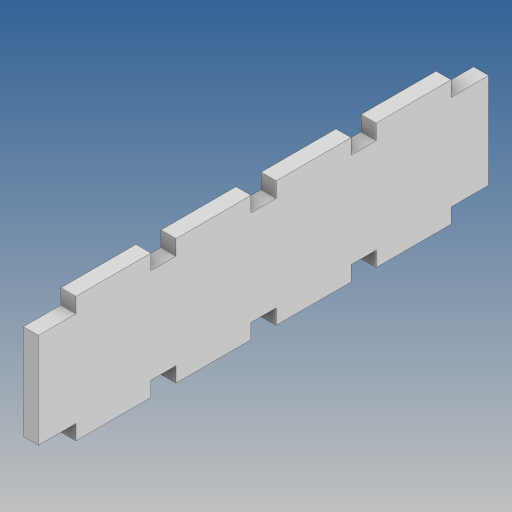
# Autodesk Inventor part: Pieza9
Saved by Autodesk Inventor 2024 (Build 280153000, 153)
## iProperties
Created: 2024-05-31
Part Number: Pieza9
Material: Genérico
Document SubType Name: Modeling
Designer: Pablo
Density: 1 g/cm^3
Appearance: Valor por defecto
Author: Pablo
Autodesk Inventor part; units mm, degrees
ref_plane "YZ Plane" through (0, 0, 0) normal (1, 0, 0) x (0, 1, 0)
ref_plane "XZ Plane" through (0, 0, 0) normal (0, 1, 0) x (-1, 0, 0)
ref_plane "XY Plane" through (0, 0, 0) normal (0, 0, 1) x (1, 0, 0)
sketch "Boceto1" plane through (0, 0, 0) normal (1, 0, 0) x (0, 1, 0)
  line L0 (0, 0) -> (19, 0)
  line L1 (19, 0) -> (19, -90)
  line L2 (19, -90) -> (0, -90)
  line L3 (0, -90) -> (0, 0)
  line L4 (19, -7.5) -> (22, -7.5)
  line L5 (22, -7.5) -> (22, -22.5)
  line L6 (22, -22.5) -> (19, -22.5)
  line L7 (19, -22.5) -> (19, -7.5)
  line L8 (19, -27.5) -> (22, -27.5)
  line L9 (22, -27.5) -> (22, -42.5)
  line L10 (22, -42.5) -> (19, -42.5)
  line L11 (19, -42.5) -> (19, -27.5)
  line L12 (19, -47.5) -> (22, -47.5)
  line L13 (22, -47.5) -> (22, -62.5)
  line L14 (22, -62.5) -> (19, -62.5)
  line L15 (19, -62.5) -> (19, -47.5)
  line L16 (19, -67.5) -> (22, -67.5)
  line L17 (22, -67.5) -> (22, -82.5)
  line L18 (22, -82.5) -> (19, -82.5)
  line L19 (19, -82.5) -> (19, -67.5)
  line L20 (9.5, 0) -> (9.5, -90) construction
  line L21 (0, -7.5) -> (-3, -7.5)
  line L22 (-3, -7.5) -> (-3, -22.5)
  line L23 (-3, -22.5) -> (0, -22.5)
  line L24 (0, -22.5) -> (0, -7.5)
  line L25 (0, -27.5) -> (-3, -27.5)
  line L26 (-3, -27.5) -> (-3, -42.5)
  line L27 (-3, -42.5) -> (0, -42.5)
  line L28 (0, -42.5) -> (0, -27.5)
  line L29 (0, -47.5) -> (-3, -47.5)
  line L30 (-3, -47.5) -> (-3, -62.5)
  line L31 (-3, -62.5) -> (0, -62.5)
  line L32 (0, -62.5) -> (0, -47.5)
  line L33 (0, -67.5) -> (-3, -67.5)
  line L34 (-3, -67.5) -> (-3, -82.5)
  line L35 (-3, -82.5) -> (0, -82.5)
  line L36 (0, -82.5) -> (0, -67.5)
  point P0 (20.5, -7.5)
  point P1 (20.5, -27.5)
  point P2 (20.5, -47.5)
  point P3 (20.5, -67.5)
  point P4 (-1.5, -7.5)
  point P5 (-1.5, -27.5)
  point P6 (-1.5, -47.5)
  point P7 (-1.5, -67.5)
  point P8 (0, -22.5)
  point P9 (0, -27.5)
  point P10 (0, -42.5)
  point P11 (0, -47.5)
  point P12 (0, -62.5)
  point P13 (0, -67.5)
  point P14 (0, -82.5)
  point P15 (19, -82.5)
  point P16 (19, -67.5)
  point P17 (19, -62.5)
  point P18 (19, -47.5)
  point P19 (19, -42.5)
  point P20 (19, -27.5)
  point P21 (19, -22.5)
  point P22 (0, -7.5)
  dimension "d0" = 19
  dimension "d1" = 90
  dimension "d2" = 3
  dimension "d3" = 15
  dimension "d4" = 7.5
  dimension "d7" = 20
  constraints: 74 end point, 20 symmetric about line, 4 parallel, 3 midpoint, 2 horizontal, 2 perpendicular, 1 point on line, 1 vertical, 27 other
  measures "d0" distance of L1.end L2.end
  measures "d1" distance of L0.end L1.end
  measures "d2" distance of L5.end L6.end
  measures "d3" distance of L4.end L5.end
  measures "d4" distance from line of point (20.5, -7.5) L0
  measures "d7" distance of L4.start L8.start
extrude "Extrusión1" add sketch "Boceto1" along normal blind 3
